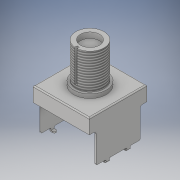
# Autodesk Inventor part: M211LW01-body-cover
Saved by Autodesk Inventor 2019 (Build 230136000, 136)
## iProperties
Created: 2022-08-22
Part Number: M211LW01-body-cover
Material: Generic
Catalog Web Link: www.cadenas.de
Description: Series M2100 - LED Tipped Actuators - body cover-
Vendor: NKKSWITCHES
Document SubType Name: Modeling
Designer: psAdmin
Manufacturer: NKKSWITCHES
Mass: 0.386082 g
Surface Area: 11.3477 cm^2
Volume: 0.386082 cm^3
Density: 1 g/cm^3
Appearance: PSOLRGB-175-175-175
Category: PARTsolutions
Company: NKKSWITCHES
Title: M211LW01-body-cover
Author: Cadenas PARTsolutions
PSOL_IDENT_0: {$CADENAS_DATA/23d-libs/nkkswitches/toggle/m2100/parts/m2100_body_cover.prj},237 {VTYP=3D},{NB=M211L
PSOL_IDENT_1: W01-body-cover},{LINA=M211LW01-body-cover},{NN=Series M2100 - LED Tipped Actuators - body cover},{DA
PSOL_IDENT_2: TE=02.08.2022 07:27:12},{GEOMDATE=24.04.2009 11:07:00},{VERSION=},{LINEID=10},{WBVAR=PLS,LCAT,CMRT,T
PSOL_IDENT_3: MT},{WBNUMERIC=}  {NB=M211LW01-body-cover},{LINA=M211LW01-body-cover},{KT=DUMMY},{PN=M211LW01},{SRS=
PSOL_IDENT_4: M21},{PLS=1},{LCAT=L},{LCAT1= 'L','L - Isolated (Toggle)','T','T - Synchronous (Toggle)','R','R - Is
PSOL_IDENT_5: olated (Rocker)','N','N - Synchronous (Rocker)','P','P - Isolated (Paddle)','J','J - Synchronous (Pa
PSOL_IDENT_6: ddle)' },{CMRT=W},{TMT=01},{TMT1= '01','01 - Solder Lug with Threaded Bushing','02','02 - Quick Conn
PSOL_IDENT_7: ect with Threaded Bushing','03','03 - Straight PC with Threaded Bushing' },{ND=0.25}
NB: M211LW01-body-cover
NN: Series M2100 - LED Tipped Actuators - body cover
NBSYN: $PN.-body-cover
LINA: M211LW01-body-cover
CATALOG: NKK Switches
PN: M211LW01
SRS: M21
PLS: 1 - SPDT
LCAT: L - Isolated (Toggle)
CMRT: W - Silver; Rated 6A @ 125V AC
TMT: 01 - Solder Lug with Threaded Bushing
SUPPLIER: NKKSWITCHES
ARTICLENO: M211LW01-body-cover
BOMINFO: M211LW01-body-cover
CREATOR: CADENAS GmbH
Autodesk Inventor part; units mm, degrees
sketch "Sketch_1" plane through (0, 0, 0) normal (1, 0, 0) x (0, 1, 0)
  line L0 (9.7536, 6.5024) -> (9.7536, 5.4864)
  arc A0 (9.2456, 4.9784) -> (9.7536, 5.4864) centre (9.2456, 5.4864) ccw
  line L1 (9.2456, 4.9784) -> (2.54, 4.9784)
  line L2 (2.54, 4.9784) -> (2.54, -4.9784)
  line L3 (2.54, -4.9784) -> (9.2456, -4.9784)
  arc A1 (9.7536, -5.4864) -> (9.2456, -4.9784) centre (9.2456, -5.4864) ccw
  line L4 (9.7536, -5.4864) -> (9.7536, -6.5024)
  line L5 (9.7536, -6.5024) -> (12.8016, -6.5024)
  arc A2 (12.8016, -6.5024) -> (13.0556, -6.2484) centre (12.8016, -6.2484) ccw
  line L6 (13.0556, -6.2484) -> (13.0556, 6.2484)
  arc A3 (13.0556, 6.2484) -> (12.8016, 6.5024) centre (12.8016, 6.2484) ccw
  line L7 (12.8016, 6.5024) -> (9.7536, 6.5024)
  constraints: 16 end point, 8 point on circle, 4 centre point
extrude "Extrusion1" add sketch "Sketch_1" along normal mid plane 12.7
sketch "Sketch_2" plane through (0, 0, 0) normal (0, 1, 0) x (-1, 0, 0)
  line L0 (6.096, 6.2484) -> (-6.096, 6.2484)
  line L1 (-6.096, 6.2484) -> (-6.096, -6.2484)
  line L2 (-6.096, -6.2484) -> (6.096, -6.2484)
  line L3 (6.096, -6.2484) -> (6.096, 6.2484)
  constraints: 8 end point
extrude "Extrusion2" cut sketch "Sketch_2" along normal blind 12.8016
sketch "Sketch_3" plane through (0, 0, 0) normal (0, 0, 1) x (1, 0, 0)
  arc A0 (-6.096, 13.0556) -> (-6.35, 12.8016) centre (-6.096, 12.8016) ccw
  line L0 (-6.096, 13.0556) -> (6.096, 13.0556)
  arc A1 (6.35, 12.8016) -> (6.096, 13.0556) centre (6.096, 12.8016) ccw
  line L1 (6.35, 12.8016) -> (6.35, 15.24)
  line L2 (6.35, 15.24) -> (-6.35, 15.24)
  line L3 (-6.35, 15.24) -> (-6.35, 12.8016)
  constraints: 8 end point, 4 point on circle, 2 centre point
extrude "Extrusion3" cut sketch "Sketch_3" along normal mid plane 25.6032
sketch "Sketch_4" plane through (0, 2.54, 0) normal (0, 1, 0) x (1, 0, 0)
  line L0 (-6.096, 5.4864) -> (-6.096, -5.4864)
  line L1 (-6.096, -5.4864) -> (-6.35, -5.4864)
  line L2 (-6.35, -5.4864) -> (-6.35, 5.4864)
  line L3 (-6.35, 5.4864) -> (-6.096, 5.4864)
  line L4 (-6.096, 5.4864) -> (-6.096, -5.4864)
  constraints: 10 end point
revolve "Revolution1" add sketch "Sketch_4" angle 90 about axis through (-6.096, 2.54, -5.4864) along (0, 0, 1)
sketch "Sketch_5" plane through (0, 2.54, 0) normal (0, 1, 0) x (1, 0, 0)
  line L0 (6.096, -5.4864) -> (6.096, 5.4864)
  line L1 (6.096, 5.4864) -> (6.35, 5.4864)
  line L2 (6.35, 5.4864) -> (6.35, -5.4864)
  line L3 (6.35, -5.4864) -> (6.096, -5.4864)
  line L4 (6.096, -5.4864) -> (6.096, 5.4864)
  constraints: 10 end point
revolve "Revolution2" add sketch "Sketch_5" angle 90 about axis through (6.096, 2.54, 5.4864) along (0, 0, -1)
sketch "Sketch_6" plane through (0, 2.54, 0) normal (0, 1, 0) x (1, 0, 0)
  line L0 (-6.096, -2.7305) -> (-5.715, -2.7305)
  arc A0 (-5.715, -2.7305) -> (-5.715, -1.9685) centre (-5.715, -2.3495) ccw
  line L1 (-5.715, -1.9685) -> (-5.715, 1.9685)
  arc A1 (-5.715, 1.9685) -> (-5.715, 2.7305) centre (-5.715, 2.3495) ccw
  line L2 (-5.715, 2.7305) -> (-6.096, 2.7305)
  line L3 (-6.096, 2.7305) -> (-6.096, -2.7305)
  constraints: 8 end point, 4 point on circle, 2 centre point
extrude "Extrusion4" add sketch "Sketch_6" against normal blind 0.254
sketch "Sketch_7" plane through (0, 2.54, 0) normal (0, 1, 0) x (1, 0, 0)
  arc A0 (5.715, -1.9685) -> (5.715, -2.7305) centre (5.715, -2.3495) ccw
  line L0 (5.715, -2.7305) -> (6.096, -2.7305)
  line L1 (6.096, -2.7305) -> (6.096, 2.7305)
  line L2 (6.096, 2.7305) -> (5.715, 2.7305)
  arc A1 (5.715, 2.7305) -> (5.715, 1.9685) centre (5.715, 2.3495) ccw
  line L3 (5.715, 1.9685) -> (5.715, -1.9685)
  constraints: 8 end point, 4 point on circle, 2 centre point
extrude "Extrusion5" add sketch "Sketch_7" against normal blind 0.254
sketch "Sketch_8" plane through (6.35, 0, 0) normal (1, 0, 0) x (0, 0, -1)
  line L0 (-7.1863, 3.302) -> (-7.1863, 0)
  line L1 (-7.1863, 0) -> (7.752, 0)
  line L2 (7.752, 0) -> (7.752, 3.302)
  line L3 (7.752, 3.302) -> (4.9784, 3.302)
  arc A0 (4.7244, 3.048) -> (4.9784, 3.302) centre (4.7244, 3.302) ccw
  line L4 (4.7244, 3.048) -> (2.9845, 3.048)
  arc A1 (2.9845, 3.048) -> (2.7305, 2.794) centre (2.9845, 2.794) ccw
  line L5 (2.7305, 2.794) -> (2.7305, 2.286)
  line L6 (2.7305, 2.286) -> (1.9685, 2.286)
  line L7 (1.9685, 2.286) -> (1.9685, 2.794)
  arc A2 (1.9685, 2.794) -> (1.7145, 3.048) centre (1.7145, 2.794) ccw
  line L8 (1.7145, 3.048) -> (-1.7145, 3.048)
  arc A3 (-1.7145, 3.048) -> (-1.9685, 2.794) centre (-1.7145, 2.794) ccw
  line L9 (-1.9685, 2.794) -> (-1.9685, 2.286)
  line L10 (-1.9685, 2.286) -> (-2.7305, 2.286)
  line L11 (-2.7305, 2.286) -> (-2.7305, 2.794)
  arc A4 (-2.7305, 2.794) -> (-2.9845, 3.048) centre (-2.9845, 2.794) ccw
  line L12 (-2.9845, 3.048) -> (-4.7244, 3.048)
  arc A5 (-4.9784, 3.302) -> (-4.7244, 3.048) centre (-4.7244, 3.302) ccw
  line L13 (-4.9784, 3.302) -> (-7.1863, 3.302)
  constraints: 28 end point, 12 point on circle, 6 centre point
extrude "Extrusion6" cut sketch "Sketch_8" against normal blind 25.4
sketch "Sketch_17" plane through (0, 0, 0) normal (0, 0, 1) x (1, 0, 0)
  line L0 (0, 13.0556) -> (0, 21.9456)
  line L1 (0, 21.9456) -> (3.175, 21.9456)
  line L2 (3.175, 21.9456) -> (3.175, 13.9446)
  line L3 (3.175, 13.9446) -> (3.683, 13.9446)
  line L4 (3.683, 13.9446) -> (3.683, 13.0556)
  line L5 (3.683, 13.0556) -> (0, 13.0556)
  line L6 (0, 13.0556) -> (0, 21.9456)
  constraints: 14 end point
revolve "Revolution3" add sketch "Sketch_17" angle 360 about axis through (0, 13.0556, 0) along (0, -1, 0)
thread "Thread1" size "1/4-48 UNS" class "2A" standard "ANSI Unified Screw Threads" full length
sketch "Sketch_19" plane through (0, 0, 0) normal (0, 0, 1) x (1, 0, 0)
  line L0 (0, 20.6756) -> (0, 21.9456)
  line L1 (0, 21.9456) -> (2.159, 21.9456)
  line L2 (2.159, 21.9456) -> (2.159, 20.6756)
  line L3 (2.159, 20.6756) -> (0, 20.6756)
  line L4 (0, 20.6756) -> (0, 21.9456)
  constraints: 10 end point
revolve "Revolution4" cut sketch "Sketch_19" angle 360 about axis through (0, 20.6756, 0) along (0, -1, 0)
sketch "Sketch_35" plane through (0, 14.7066, 0) normal (0, 1, 0) x (1, 0, 0)
  line L0 (-0.254, -2.6518) -> (-0.254, -3.175)
  line L1 (-0.254, -3.175) -> (0.254, -3.175)
  line L2 (0.254, -3.175) -> (0.254, -2.6518)
  line L3 (0.254, -2.6518) -> (-0.254, -2.6518)
  constraints: 8 end point
extrude "Extrusion7" cut sketch "Sketch_35" along normal blind 20.32
ref_plane "at507h_XY" through (0, 16.3576, 0) normal (0, 1, 0) x (1, 0, 0)
ref_plane "at507h_YZ" through (0, 16.3576, 0) normal (1, 0, 0) x (0, 0, -1)
ref_plane "at507h_ZX" through (0, 16.3576, 0) normal (0, 0, -1) x (0, 1, 0)
ref_plane "at507h_dual_XY" through (-2.4003, 16.3576, 0) normal (0, 1, 0) x (1, 0, 0)
ref_plane "at507h_dual_YZ" through (-2.4003, 16.3576, 0) normal (1, 0, 0) x (0, 0, -1)
ref_plane "at507h_dual_ZX" through (-2.4003, 16.3576, 0) normal (0, 0, -1) x (0, 1, 0)
ref_plane "at509_XY" through (0, 15.7099, 0) normal (0, 1, 0) x (1, 0, 0)
ref_plane "at509_YZ" through (0, 15.7099, 0) normal (1, 0, 0) x (0, 0, -1)
ref_plane "at509_ZX" through (0, 15.7099, 0) normal (0, 0, -1) x (0, 1, 0)
ref_plane "at509_dual_XY" through (-2.4003, 15.7099, 0) normal (0, 1, 0) x (1, 0, 0)
ref_plane "at509_dual_YZ" through (-2.4003, 15.7099, 0) normal (1, 0, 0) x (0, 0, -1)
ref_plane "at509_dual_ZX" through (-2.4003, 15.7099, 0) normal (0, 0, -1) x (0, 1, 0)
ref_plane "at513h_XY" through (0, 14.7066, 0) normal (0, 1, 0) x (1, 0, 0)
ref_plane "at513h_YZ" through (0, 14.7066, 0) normal (1, 0, 0) x (0, 0, -1)
ref_plane "at513h_ZX" through (0, 14.7066, 0) normal (0, 0, -1) x (0, 1, 0)
ref_plane "at513h_dual_XY" through (-2.4003, 14.7066, 0) normal (0, 1, 0) x (1, 0, 0)
ref_plane "at513h_dual_YZ" through (-2.4003, 14.7066, 0) normal (1, 0, 0) x (0, 0, -1)
ref_plane "at513h_dual_ZX" through (-2.4003, 14.7066, 0) normal (0, 0, -1) x (0, 1, 0)
ref_plane "body_c_to_bracket_XY" through (0, 13.0556, 0) normal (0, -1, 0) x (1, 0, 0)
ref_plane "body_c_to_bracket_YZ" through (0, 13.0556, 0) normal (1, 0, 0) x (0, 0, 1)
ref_plane "body_c_to_bracket_ZX" through (0, 13.0556, 0) normal (0, 0, 1) x (0, -1, 0)
ref_plane "body_cover_to_body_XY" through (0, 12.8016, 0) normal (0, 1, 0) x (1, 0, 0)
ref_plane "body_cover_to_body_YZ" through (0, 12.8016, 0) normal (1, 0, 0) x (0, 0, -1)
ref_plane "body_cover_to_body_ZX" through (0, 12.8016, 0) normal (0, 0, -1) x (0, 1, 0)
ref_plane "body_cover_to_toggle_XY" through (0, 18.1356, 0) normal (0, 1, 0) x (1, 0, 0)
ref_plane "body_cover_to_toggle_YZ" through (0, 18.1356, 0) normal (1, 0, 0) x (0, 0, -1)
ref_plane "body_cover_to_toggle_ZX" through (0, 18.1356, 0) normal (0, 0, -1) x (0, 1, 0)
ref_plane "body_cover_to_toggle2_XY" through (-2.4003, 18.1356, 0) normal (0, 1, 0) x (1, 0, 0)
ref_plane "body_cover_to_toggle2_YZ" through (-2.4003, 18.1356, 0) normal (1, 0, 0) x (0, 0, -1)
ref_plane "body_cover_to_toggle2_ZX" through (-2.4003, 18.1356, 0) normal (0, 0, -1) x (0, 1, 0)
ref_plane "st513h_2_XY" through (0, 17.5006, 0) normal (0, 1, 0) x (1, 0, 0)
ref_plane "st513h_2_YZ" through (0, 17.5006, 0) normal (1, 0, 0) x (0, 0, -1)
ref_plane "st513h_2_ZX" through (0, 17.5006, 0) normal (0, 0, -1) x (0, 1, 0)
ref_plane "st513h_2_dual_XY" through (-2.4003, 17.5006, 0) normal (0, 1, 0) x (1, 0, 0)
ref_plane "st513h_2_dual_YZ" through (-2.4003, 17.5006, 0) normal (1, 0, 0) x (0, 0, -1)
ref_plane "st513h_2_dual_ZX" through (-2.4003, 17.5006, 0) normal (0, 0, -1) x (0, 1, 0)
body "Solid1"
